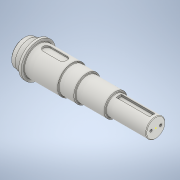
# Autodesk Inventor part: 轴
Saved by Autodesk Inventor 2020 (Build 240168000, 168)
## iProperties
CustomPartVersion: 1
Created: 2021-06-09
Part Number: 轴
Material: Steel
Document SubType Name: Modeling
Designer: dell
Density: 1 g/cm^3
Appearance: Steel
Length: 579.000 mm
Author: dell
Autodesk Inventor part; units mm, degrees
ref_plane "起始平面" through (0, 0, 0) normal (1, 0, 0) x (0, 1, 0)
sketch "主草图" plane through (0, 0, 0) normal (0, 0, 1) x (1, 0, 0)
  line L0 (0, 0) -> (579, 0)
  line L1 (0, 0) -> (0, 55)
  line L2 (0, 55) -> (50, 55)
  line L3 (50, 55) -> (50, 58)
  line L4 (50, 58) -> (79, 58)
  line L5 (79, 58) -> (79, 72)
  line L6 (89, 72) -> (89, 60)
  line L7 (79, 72) -> (89, 72)
  line L8 (229, 60) -> (229, 55)
  line L9 (89, 60) -> (229, 60)
  line L10 (311, 55) -> (311, 48)
  line L11 (229, 55) -> (311, 55)
  line L12 (411, 48) -> (411, 40)
  line L13 (311, 48) -> (411, 48)
  line L14 (579, 40) -> (579, 0)
  line L15 (411, 40) -> (579, 40)
  dimension "d3" = 110
  dimension "d4" = 116
  dimension "d5" = 144
  dimension "d6" = 120
  dimension "d7" = 110
  dimension "d8" = 96
  dimension "d9" = 80
  constraints: 32 end point, 8 vertical, 2 horizontal
  measures "d3" diameter of L2 L0
  measures "d4" diameter of L4 L0
  measures "d5" diameter of L7 L0
  measures "d6" diameter of L9 L0
  measures "d7" diameter of L11 L0
  measures "d8" diameter of L13 L0
  measures "d9" diameter of L15 L0
revolve "旋转1" add sketch "主草图" angle 360 about axis through (0, 0, 0) along (1, 0, 0)
sketch "草图6" plane through (311, 0, 0) normal (1, 0, 0) x (0, 0, -1)
  circle A0 centre (0, 0) radius 48 projected
  circle A1 centre (0, 0) radius 48 projected
  circle A2 centre (0, 0) radius 55 projected
extrude "拉伸4" cut sketch "草图6" against normal blind 19
sketch "草图7" plane through (0, 0, 0) normal (-1, 0, 0) x (0, 0, 1)
  circle A0 centre (0, 0) radius 55 projected
extrude "拉伸5" cut sketch "草图7" against normal blind 30
chamfer "倒角1" distance 2.5 angle 45 2 edges at (579, -40, 0) (30, -55, 0)
fillet "圆角1" radius 2 6 edges at (411, -40, 0) (292, 0, 48) (229, -55, 0) (89, -60, 0) (79, -58, 0) (50, -55, 0)
sketch "草图8" plane through (579, 0, 0) normal (1, 0, 0) x (0, 0, -1)
  point P0 (0, 0)
sketch "草图9" plane through (579, 0, 0) normal (1, 0, 0) x (0, 0, -1)
  line L0 (-100.8, 0) -> (100.8, 0) construction
  line L1 (0, -100.8) -> (0, 100.8) construction
  point P0 (0, 0)
  point P1 (20, 0)
  point P2 (-20, 0)
  dimension "d28" = 40
  constraints: 2 point on line, 1 symmetric about line
  measures "d28" distance of point (-20, 0) point (20, 0)
hole "孔1" at (579, 0, -20) at (579, 0, 20) direction (-1, 0, 0) diameter 10.106 depth 25 tip angle 118 thread size "M12x1.75" designation "M12" class "6H" standard "GB Metric profile"
ref_plane "工作平面1" through (495, 40, 0) normal (0, 1, 0) x (-1, 0, 0)
sketch "草图10" plane through (495, 40, 0) normal (0, 1, 0) x (-1, 0, 0)
  line L0 (-199.8, 0) -> (610.8, 0) construction
  line L1 (84, -48) -> (84, 48) construction
  line L2 (-84, -37.5) -> (-84, 37.5) construction
  line L3 (70, -11) -> (-70, -11)
  line L4 (-70, -11) -> (-70, 11)
  line L5 (-70, 11) -> (70, 11)
  line L6 (70, 11) -> (70, -11)
  point P0 (495, 0)
  dimension "d36" = 140
  dimension "d37" = 22
  dimension "d38" = 14
  constraints: 8 end point, 2 parallel, 1 horizontal, 1 perpendicular, 1 other
  measures "d36" distance of L4.end L5.end
  measures "d37" distance of L3.end L4.end
  measures "d38" distance between parallel lines of L2 L4
extrude "拉伸6" cut sketch "草图10" against normal blind 9
ref_plane "工作平面2" through (159, 60, 0) normal (0, 1, 0) x (-1, 0, 0)
sketch "草图11" plane through (159, 60, 0) normal (0, 1, 0) x (-1, 0, 0)
  line L0 (34, 0) -> (-34, 0) construction
  line L1 (34, 16) -> (-34, 16)
  line L2 (-34, -16) -> (34, -16)
  arc A0 (34, -16) -> (34, 16) centre (34, 0) ccw
  arc A1 (-34, 16) -> (-34, -16) centre (-34, 0) ccw
  line L3 (-535.8, 0) -> (274.8, 0) construction
  line L4 (70, -72) -> (70, 72) projected
  line L5 (-70, -60) -> (-70, 60) projected
  point P0 (159, 0)
  point P1 (0, 0)
  dimension "d41" = 100
  dimension "d42" = 32
  dimension "d43" = 36
  constraints: 8 end point, 4 point on circle, 4 tangent, 2 centre point, 1 horizontal, 1 midpoint, 1 parallel, 1 other
  measures "d42" distance between parallel lines of L1 L2
  measures "d43" distance from line of L5 L0.end
extrude "拉伸7" cut sketch "草图11" against normal blind 7
equation "\"Length\" = 579"
